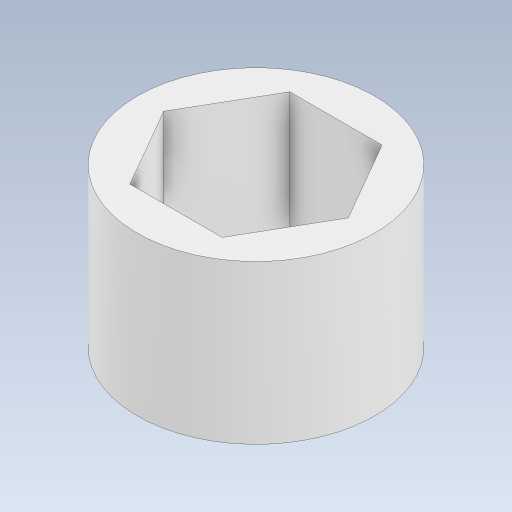
# Autodesk Inventor part: INDX_008_0.5inSpacer
Saved by Autodesk Inventor 2024 (Build 280153000, 153)
## iProperties
Created: 2024-08-09
Part Number: INDX_008_0.5inSpacer
Material: ABS Plastic
Document SubType Name: Modeling
Designer: Oscar
Density: 1.06 g/cm^3
Appearance: Smooth - White
Author: Oscar
Autodesk Inventor part; units mm, degrees
ref_plane "YZ Plane" through (0, 0, 0) normal (1, 0, 0) x (0, 1, 0)
ref_plane "XZ Plane" through (0, 0, 0) normal (0, 1, 0) x (-1, 0, 0)
ref_plane "XY Plane" through (0, 0, 0) normal (0, 0, 1) x (1, 0, 0)
sketch "Sketch1" plane through (0, 0, 0) normal (0, 1, 0) x (-1, 0, 0)
  circle A0 centre (0, 0) radius 9.525
  line L0 (-3.7028, 6.4135) -> (3.7028, 6.4135)
  line L1 (3.7028, 6.4135) -> (7.4057, 0)
  line L2 (7.4057, 0) -> (3.7028, -6.4135)
  line L3 (3.7028, -6.4135) -> (-3.7028, -6.4135)
  line L4 (-3.7028, -6.4135) -> (-7.4057, 0)
  line L5 (-7.4057, 0) -> (-3.7028, 6.4135)
  dimension "d0" = 19.05
  dimension "d1" = 12.827
  constraints: 12 end point, 2 coincident, 1 centre point, 1 horizontal, 13 other
  measures "d0" diameter of A0
  measures "d1" distance between parallel lines of L3 L0
extrude "Extrusion1" add sketch "Sketch1" along normal blind 12.7
body "Solid1"
